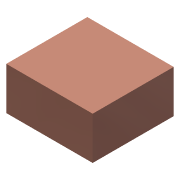
# Autodesk Inventor part: LIPO
Saved by Autodesk Inventor 2017 (Build 210142000, 142)
## iProperties
Part Number: LIPO
Material: Generisch
Document SubType Name: Modeling
Designer: Werkstatt
Density: 1 g/cm^3
Appearance: JST-2-SMD, LIPO
Author: Werkstatt
Autodesk Inventor part; units mm, degrees
ref_plane "YZ Plane" through (0, 0, 0) normal (1, 0, 0) x (0, 1, 0)
ref_plane "XZ Plane" through (0, 0, 0) normal (0, 1, 0) x (-1, 0, 0)
ref_plane "XY Plane" through (0, 0, 0) normal (0, 0, 1) x (1, 0, 0)
sketch "JST-2-SMD, LIPO_23" plane through (0, 0, 0) normal (0, 0, 1) x (1, 0, 0)
  line L0 (-4.1016, 3) -> (4, 3)
  line L1 (4, 3) -> (4, -4.6016)
  line L2 (4, -4.6016) -> (-4.1016, -4.6016)
  line L3 (-4.1016, -4.6016) -> (-4.1016, 3)
  constraints: 8 end point
extrude "Extrusion1" add sketch "JST-2-SMD, LIPO_23" along normal blind 4
